Autodesk Fusion 360 part; units mm, degrees
(part 6 of 7)
  line L382 (70.9, -77.2) -> (47.4908, -77.2)
  arc A190 (46.4092, -77.2) -> (47.4908, -77.2) centre (46.95, -80.1) ccw
  line L383 (46.4092, -77.2) -> (23, -77.2)
  line L384 (23, -77.2) -> (23, -81.15)
  arc A191 (18, -81.15) -> (23, -81.15) centre (20.5, -81.15) ccw
  line L385 (27.2, 4.5) -> (27.2, 33.9)
  line L386 (27.2, 33.9) -> (66.7, 33.9)
  line L387 (66.7, 33.9) -> (66.7, 4.5)
  line L388 (66.7, 4.5) -> (27.2, 4.5)
  arc A192 (28.2, 12.5) -> (31.2, 9.5) centre (31.2, 12.5) ccw
  line L389 (31.2, 9.5) -> (62.7, 9.5)
  arc A193 (62.7, 9.5) -> (65.7, 12.5) centre (62.7, 12.5) ccw
  line L390 (65.7, 12.5) -> (65.7, 25.9)
  arc A194 (65.7, 25.9) -> (62.7, 28.9) centre (62.7, 25.9) ccw
  line L391 (62.7, 28.9) -> (31.2, 28.9)
  arc A195 (31.2, 28.9) -> (28.2, 25.9) centre (31.2, 25.9) ccw
  line L392 (28.2, 25.9) -> (28.2, 12.5)
  line L393 (-2, -85.1) -> (106.4, -85.1)
  line L394 (106.4, -85.1) -> (75.9, -85.1)
  line L395 (75.9, -85.1) -> (-2, -85.1)
  line L396 (24.5, -83.65) -> (24.5, -81.15)
  line L397 (24.5, -81.15) -> (24.5, -77.2)
  line L398 (24.5, -77.2) -> (16.5, -77.2)
  line L399 (16.5, -77.2) -> (16.5, -83.65)
  line L400 (16.5, -83.65) -> (-2, -83.65)
  line L401 (-2, -83.65) -> (-2, -3.65)
  line L402 (-2, -3.65) -> (-7, -3.65)
  line L403 (-7, -3.65) -> (-7, 4.1)
  line L404 (-7, 4.1) -> (100.9, 4.1)
  line L405 (100.9, 4.1) -> (100.9, -3.65)
  line L406 (100.9, -3.65) -> (95.9, -3.65)
  line L407 (95.9, -3.65) -> (95.9, -83.65)
  line L408 (95.9, -83.65) -> (24.5, -83.65)
  circle A196 centre (10.06, -44.3) radius 2.5
  circle A197 centre (8, -81.15) radius 1
  circle A198 centre (80.15, -44.4) radius 2.5
  circle A199 centre (-4.5, 1.6) radius 1
  circle A200 centre (73.4, -81.15) radius 1
  circle A201 centre (98.4, 1.6) radius 1
  circle A202 centre (84.4, -5) radius 2.5
  line L409 (16.5, -83.65) -> (-2, -83.65)
  line L410 (-2, -83.65) -> (16.5, -83.65)
  line L411 (27.2, 4.5) -> (66.7, 4.5)
  line L412 (66.7, 4.5) -> (27.2, 4.5)
  line L413 (16.5, -77.2) -> (16.5, -83.65)
  line L414 (16.5, -83.65) -> (16.5, -77.2)
  line L415 (116.4, 35.3) -> (-22.5, 35.3)
  line L416 (-22.5, 35.3) -> (-2.5, 35.3)
  line L417 (-2.5, 35.3) -> (96.4, 35.3)
  line L418 (96.4, 35.3) -> (116.4, 35.3)
  circle A203 centre (10.06, -44.3) radius 2.5
  circle A204 centre (10.06, -44.3) radius 2.5
  line L419 (96.4, 34.3) -> (96.4, 35.3)
  line L420 (96.4, 35.3) -> (-2.5, 35.3)
  line L421 (-2.5, 35.3) -> (-2.5, 34.3)
  line L422 (-2.5, 34.3) -> (-22.5, 34.3)
  arc A205 (-22.5, 34.3) -> (-31.5, 25.3) centre (-22.5, 25.3) ccw
  line L423 (-31.5, 25.3) -> (-31.5, 4.1)
  line L424 (-31.5, 4.1) -> (-25, 4.1)
  line L425 (-25, 4.1) -> (-25, 1.6)
  arc A206 (-23, 4.0495) -> (-25, 1.6) centre (-22.5, 1.6) ccw
  line L426 (-23, 4.0495) -> (-23, 22.8505)
  arc A207 (-22, 22.8505) -> (-23, 22.8505) centre (-22.5, 25.3) ccw
  line L427 (-22, 22.8505) -> (-22, 4.0495)
  arc A208 (-20, 1.6) -> (-22, 4.0495) centre (-22.5, 1.6) ccw
  line L428 (-20, 1.6) -> (-20, 2)
  line L429 (-20, 2) -> (-7, 2)
  line L430 (-7, 2) -> (-7, 4.1)
  line L431 (-7, 4.1) -> (-4.5, 4.1)
  line L432 (-4.5, 4.1) -> (-2, 4.1)
  line L433 (-2, 4.1) -> (0, 4.1)
  line L434 (0, 4.1) -> (0, 5.7)
  arc A209 (13.4164, 23.7) -> (0, 5.7) centre (0, 19.7) ccw
  line L435 (13.4164, 23.7) -> (27.2, 23.7)
  line L436 (27.2, 23.7) -> (27.2, 33.9)
  line L437 (27.2, 33.9) -> (66.7, 33.9)
  line L438 (66.7, 33.9) -> (66.7, 23.7)
  line L439 (66.7, 23.7) -> (80.4836, 23.7)
  arc A210 (93.9, 5.7) -> (80.4836, 23.7) centre (93.9, 19.7) ccw
  line L440 (93.9, 5.7) -> (93.9, 4.1)
  line L441 (93.9, 4.1) -> (95.9, 4.1)
  line L442 (95.9, 4.1) -> (98.4, 4.1)
  line L443 (98.4, 4.1) -> (100.9, 4.1)
  line L444 (100.9, 4.1) -> (100.9, 2)
  line L445 (100.9, 2) -> (113.9322, 2)
  arc A211 (115.9, 4.0495) -> (113.9322, 2) centre (116.4, 1.6) ccw
  line L446 (115.9, 4.0495) -> (115.9, 22.8505)
  arc A212 (116.9, 22.8505) -> (115.9, 22.8505) centre (116.4, 25.3) ccw
  line L447 (116.9, 22.8505) -> (116.9, 4.0495)
  arc A213 (118.9, 1.6) -> (116.9, 4.0495) centre (116.4, 1.6) ccw
  line L448 (118.9, 1.6) -> (118.9, 4.1)
  line L449 (118.9, 4.1) -> (125.4, 4.1)
  line L450 (125.4, 4.1) -> (125.4, 25.3)
  arc A214 (125.4, 25.3) -> (116.4, 34.3) centre (116.4, 25.3) ccw
  line L451 (116.4, 34.3) -> (96.4, 34.3)
  line L452 (-2, -3.65) -> (-2, -83.65)
  line L453 (-2, -83.65) -> (-2, -3.65)
  line L454 (24.5, -81.15) -> (24.5, -77.2)
  line L455 (24.5, -77.2) -> (24.5, -81.15)
  line L456 (-12.5, -85.1) -> (-12.5, -84.1)
  line L457 (-12.5, -84.1) -> (106.4, -84.1)
  line L458 (106.4, -85.1) -> (106.4, -84.1)
  line L459 (106.4, -85.1) -> (-2, -85.1)
  line L460 (-2, -85.1) -> (-12.5, -85.1)
  line L461 (66.7, 33.9) -> (27.2, 33.9)
  line L462 (27.2, 33.9) -> (66.7, 33.9)
  circle A215 centre (-4.5, 1.6) radius 1
  circle A216 centre (-4.5, 1.6) radius 1
  arc A217 (83.1181, 15.7) -> (83.1181, 23.7) centre (93.9, 19.7) ccw
  line L463 (83.1181, 23.7) -> (66.7, 23.7)
  line L464 (66.7, 23.7) -> (66.7, 15.7)
  line L465 (66.7, 15.7) -> (83.1181, 15.7)
  arc A218 (102.9, 18.7) -> (102.9, 20.7) centre (102.9, 19.7) ccw
  line L466 (102.9, 18.7) -> (84.9, 18.7)
  arc A219 (84.9, 20.7) -> (84.9, 18.7) centre (84.9, 19.7) ccw
  line L467 (84.9, 20.7) -> (102.9, 20.7)
  arc A220 (98.9004, 26.7) -> (98.9, 28.7) centre (98.9, 27.7) ccw
  line L468 (98.9004, 26.7) -> (88.8996, 26.7)
  arc A221 (88.9, 28.7) -> (88.8996, 26.7) centre (88.9, 27.7) ccw
  line L469 (88.9, 28.7) -> (98.9, 28.7)
  arc A222 (102.0652, 22.7) -> (102.0652, 24.7) centre (102.0652, 23.7) ccw
  line L470 (102.0652, 22.7) -> (85.7348, 22.7)
  arc A223 (85.7348, 24.7) -> (85.7348, 22.7) centre (85.7348, 23.7) ccw
  line L471 (85.7348, 24.7) -> (102.0652, 24.7)
  line L472 (102.0652, 14.7) -> (85.7348, 14.7)
  arc A224 (85.7348, 16.7) -> (85.7348, 14.7) centre (85.7348, 15.7) ccw
  line L473 (85.7348, 16.7) -> (102.0652, 16.7)
  arc A225 (102.0652, 14.7) -> (102.0652, 16.7) centre (102.0652, 15.7) ccw
  line L474 (88.8996, 12.7) -> (98.8996, 12.7)
  arc A226 (98.9, 10.7) -> (98.8996, 12.7) centre (98.9, 11.7) ccw
  line L475 (98.9, 10.7) -> (88.9, 10.7)
  arc A227 (88.8996, 12.7) -> (88.9, 10.7) centre (88.9, 11.7) ccw
  line L476 (-23.188, -62.3239) -> (-23.188, -59.3239)
  arc A228 (-20.188, -59.3239) -> (-23.188, -59.3239) centre (-21.688, -59.3239) ccw
  line L477 (-20.188, -59.3239) -> (-20.188, -62.3239)
  arc A229 (-23.188, -62.3239) -> (-20.188, -62.3239) centre (-21.688, -62.3239) ccw
  circle A230 centre (-10.8119, -62.3239) radius 1.5
  line L478 (-2, -24.9) -> (-8, -24.9)
  line L479 (-8, -24.9) -> (-8, -7.9)
  line L480 (-8, -7.9) -> (-13, -7.9)
  line L481 (-13, -7.9) -> (-13, -13.9)
  line L482 (-13, -13.9) -> (-25, -13.9)
  line L483 (-25, -13.9) -> (-25, -24.9)
  line L484 (-25, -24.9) -> (-30.5, -24.9)
  line L485 (-30.5, -24.9) -> (-30.5, -25.9)
  line L486 (-30.5, -25.9) -> (-31.5, -25.9)
  line L487 (-31.5, -25.9) -> (-31.5, 4.1)
  line L488 (-31.5, 4.1) -> (-32.5, 4.1)
  line L489 (-32.5, 4.1) -> (-32.5, -25.2)
  line L490 (-32.5, -25.2) -> (-32.5, -65.1)
  arc A231 (-32.5, -65.1) -> (-12.5, -85.1) centre (-12.5, -65.1) ccw
  line L491 (-12.5, -85.1) -> (-2, -85.1)
  line L492 (-2, -85.1) -> (-2, -24.9)
  arc A232 (-9.5307, -48.3426) -> (-9.5307, -34.5574) centre (-10.1676, -41.45) ccw
  arc A233 (-22.9827, -48.1827) -> (-9.5307, -48.3426) centre (-16.25, -47.7) ccw
  arc A234 (-22.9827, -34.7173) -> (-22.9827, -48.1827) centre (-22.5, -41.45) ccw
  arc A235 (-9.5307, -34.5574) -> (-22.9827, -34.7173) centre (-16.25, -35.2) ccw
  circle A236 centre (-16.25, -62.1) radius 2.5
  line L493 (-14, -21.7213) -> (-14, -21.5571)
  arc A237 (-18.6299, -19.9) -> (-14, -21.5571) centre (-16.1626, -20.3028) ccw
  line L494 (-18.6299, -19.9) -> (-18.6563, -19.9)
  arc A238 (-18.6098, -19.7916) -> (-18.6563, -19.9) centre (-16.3363, -20.8316) ccw
  arc A239 (-13.8891, -21.3427) -> (-18.6098, -19.7916) centre (-16.1626, -20.3028) ccw
  arc A240 (-14, -21.7213) -> (-13.8891, -21.3427) centre (-16.3363, -20.8316) ccw
  line L495 (-28.5, -61.1) -> (-28.5, -52.1)
  line L496 (-28.5, -52.1) -> (-27.5, -52.1)
  line L497 (-27.5, -52.1) -> (-27.5, -62.1)
  line L498 (-27.5, -62.1) -> (-24.5, -65.1)
  line L499 (-24.5, -65.1) -> (-19.8023, -65.1)
  arc A241 (-19.8023, -65.1) -> (-12.5, -72.4023) centre (-12.5, -65.1) ccw
  line L500 (-12.5, -72.4023) -> (-12.5, -77.1)
  line L501 (-12.5, -77.1) -> (-6.5, -83.1)
  line L502 (-6.5, -83.1) -> (-6.5, -84.1)
  line L503 (-6.5, -84.1) -> (-12.5, -84.1)
  arc A242 (-31.5, -65.1) -> (-12.5, -84.1) centre (-12.5, -65.1) ccw
  line L504 (-31.5, -65.1) -> (-31.5, -59.1)
  line L505 (-31.5, -59.1) -> (-30.5, -59.1)
  line L506 (-30.5, -59.1) -> (-28.5, -61.1)
  line L507 (-5, -57) -> (-5, -75)
  line L508 (-5, -75) -> (-6, -75)
  line L509 (-6, -75) -> (-6, -57)
  line L510 (-6, -57) -> (-5, -57)
  line L511 (-2, -71.1) -> (-2, -27.1)
  line L512 (-2, -27.1) -> (-2, -0.9)
  line L513 (-2, -0.9) -> (-2, -1.9)
  line L514 (-2, -1.9) -> (-2, -6.9)
  line L515 (-2, -6.9) -> (-2, -7.9)
  line L516 (-2, -7.9) -> (-2, -12.9)
  line L517 (-2, -12.9) -> (-2, -13.9)
  line L518 (-2, -13.9) -> (-2, -18.9)
  line L519 (-2, -18.9) -> (-2, -24.9)
  line L520 (-2, -24.9) -> (-2, -85.1)
  line L521 (-2, -85.1) -> (-2, -77.2)
  line L522 (-2, -77.2) -> (-2, -71.1)
  line L523 (-32.5, -25.2) -> (-31.5, -25.2)
  line L524 (-32.5, -25.2) -> (-32.5, 4.1)
  line L525 (-32.5, 4.1) -> (-32.5, 25.3)
  line L526 (-32.5, 25.3) -> (-31.5, 25.3)
  line L527 (-31.5, 25.3) -> (-31.5, -25.2)
  line L528 (31.2, 9.5) -> (62.7, 9.5)
  line L529 (62.7, 9.5) -> (31.2, 9.5)
  spline S8 degree 3 poles (-32.8222, -7.2428) (-33.1865, -8.6078) (-33.3665, -10.0329) (-33.3734, -12.8887) (-33.1935, -14.3424) (-32.8222, -15.7336) knots 0 0 0 0 0.423819 0.423819 0.855786 0.855786 0.855786 0.855786
  spline S9 degree 3 poles (-32.5, -4.7455) (-32.5, -5.4939) (-32.584, -6.2471) (-32.7761, -7.0646) (-32.7985, -7.1539) (-32.8222, -7.2428) knots 0 0 0 0 0.224513 0.224513 0.252112 0.252112 0.252112 0.252112
  line L530 (-32.5, -4.7455) -> (-32.5, 4.1)
  line L531 (-32.5, 4.1) -> (-31.5, 4.1)
  line L532 (-31.5, 4.1) -> (-31.5, -25.9)
  line L533 (-31.5, -25.9) -> (-31.5, -59.1)
  line L534 (-31.5, -59.1) -> (-31.5, -65.1)
  line L535 (-31.5, -65.1) -> (-32.5, -65.1)
  line L536 (-32.5, -65.1) -> (-32.5, -25.2)
  line L537 (-32.5, -25.2) -> (-32.5, -18.2308)
  spline S10 degree 3 poles (-32.8222, -15.7336) (-32.7995, -15.8187) (-32.778, -15.9042) (-32.5849, -16.7214) (-32.5, -17.4786) (-32.5, -18.2308) knots 0.187001 0.187001 0.187001 0.187001 0.213353 0.213353 0.43842 0.43842 0.43842 0.43842
  arc A243 (85.2397, 8.7) -> (93.9, 5.7) centre (93.9, 19.7) ccw
  line L538 (85.2397, 8.7) -> (66.7, 8.7)
  line L539 (66.7, 8.7) -> (66.7, 4.1)
  line L540 (66.7, 4.1) -> (93.9, 4.1)
  line L541 (93.9, 4.1) -> (93.9, 5.7)
  line L542 (-7, 4.1) -> (-7, -3.65)
  line L543 (-7, -3.65) -> (-7, 4.1)
  line L544 (-31.5, -25.9) -> (-31.5, 4.1)
  line L545 (-31.5, 4.1) -> (-31.5, -65.1)
  line L546 (-31.5, -65.1) -> (-31.5, -59.1)
  line L547 (-31.5, -59.1) -> (-31.5, -25.9)
  arc A244 (80.4836, 15.7) -> (85.2397, 8.7) centre (93.9, 19.7) ccw
  arc A245 (85.2397, 8.7) -> (93.9, 5.7) centre (93.9, 19.7) ccw
  arc A246 (93.9, 5.7) -> (80.4836, 23.7) centre (93.9, 19.7) ccw
  arc A247 (80.4836, 15.7) -> (80.4836, 23.7) centre (93.9, 19.7) ccw
  line L548 (-32.5, -18.2308) -> (-32.5, 11.7692)
  line L549 (-32.5, -18.2308) -> (-32.5, -25.2)
  line L550 (-32.5, -25.2) -> (-32.5, 11.7692)
  spline S11 degree 3 poles (-32.8222, 14.2664) (-33.1865, 15.6314) (-33.3665, 17.0565) (-33.3734, 19.9123) (-33.1935, 21.3661) (-32.8222, 22.7572) knots 0 0 0 0 0.423819 0.423819 0.855786 0.855786 0.855786 0.855786
  spline S12 degree 3 poles (-32.5, 11.7692) (-32.5, 12.5174) (-32.584, 13.2705) (-32.776, 14.088) (-32.7984, 14.1774) (-32.8222, 14.2664) knots 0 0 0 0 0.224479 0.224479 0.252112 0.252112 0.252112 0.252112
  line L551 (-32.5, 11.7692) -> (-32.5, -25.2)
  line L552 (-32.5, -25.2) -> (-32.5, -65.1)
  line L553 (-32.5, -65.1) -> (-31.5, -65.1)
  line L554 (-31.5, -65.1) -> (-31.5, 4.1)
  line L555 (-31.5, 4.1) -> (-31.5, 25.3)
  arc A248 (-22.5, 34.3) -> (-31.5, 25.3) centre (-22.5, 25.3) ccw
  line L556 (-22.5, 34.3) -> (-2.5, 34.3)
  line L557 (-2.5, 34.3) -> (-2.5, 35.3)
  line L558 (-2.5, 35.3) -> (-22.5, 35.3)
  arc A249 (-22.5, 35.3) -> (-32.5, 25.3) centre (-22.5, 25.3) ccw
  line L559 (-32.5, 25.3) -> (-32.5, 25.2545)
  spline S13 degree 3 poles (-32.8222, 22.7572) (-32.7994, 22.8424) (-32.7779, 22.928) (-32.5849, 23.7452) (-32.5, 24.5023) (-32.5, 25.2545) knots 0.187001 0.187001 0.187001 0.187001 0.213377 0.213377 0.43842 0.43842 0.43842 0.43842
  line L560 (100.9, -3.65) -> (100.9, 4.1)
  line L561 (100.9, 4.1) -> (100.9, -3.65)
  line L562 (95.9, -3.65) -> (100.9, -3.65)
  line L563 (100.9, -3.65) -> (95.9, -3.65)
  line L564 (80.4836, 23.7) -> (66.7, 23.7)
  line L565 (66.7, 23.7) -> (83.1181, 23.7)
  line L566 (83.1181, 23.7) -> (80.4836, 23.7)
  arc A250 (10.7819, 23.7) -> (10.7819, 15.7) centre (0, 19.7) ccw
  line L567 (10.7819, 15.7) -> (27.2, 15.7)
  line L568 (27.2, 15.7) -> (27.2, 23.7)
  line L569 (27.2, 23.7) -> (10.7819, 23.7)
  arc A251 (-5.0004, 12.7) -> (-5, 10.7) centre (-5, 11.7) ccw
  line L570 (-5.0004, 12.7) -> (5.0004, 12.7)
  arc A252 (5, 10.7) -> (5.0004, 12.7) centre (5, 11.7) ccw
  line L571 (5, 10.7) -> (-5, 10.7)
  arc A253 (-5, 28.7) -> (-5.0004, 26.7) centre (-5, 27.7) ccw
  line L572 (-5, 28.7) -> (5, 28.7)
  arc A254 (4.9996, 26.7) -> (5, 28.7) centre (5, 27.7) ccw
  line L573 (4.9996, 26.7) -> (-5.0004, 26.7)
  line L574 (-8.1652, 24.7) -> (8.1652, 24.7)
  arc A255 (8.1652, 22.7) -> (8.1652, 24.7) centre (8.1652, 23.7) ccw
  line L575 (8.1652, 22.7) -> (-8.1652, 22.7)
  arc A256 (-8.1652, 24.7) -> (-8.1652, 22.7) centre (-8.1652, 23.7) ccw
  line L576 (8.1652, 14.7) -> (-8.1652, 14.7)
  arc A257 (-8.1652, 16.7) -> (-8.1652, 14.7) centre (-8.1652, 15.7) ccw
  line L577 (-8.1652, 16.7) -> (8.1652, 16.7)
  arc A258 (8.1652, 14.7) -> (8.1652, 16.7) centre (8.1652, 15.7) ccw
  arc A259 (9, 18.7) -> (9, 20.7) centre (9, 19.7) ccw
  line L578 (9, 18.7) -> (-9, 18.7)
  arc A260 (-9, 20.7) -> (-9, 18.7) centre (-9, 19.7) ccw
  line L579 (-9, 20.7) -> (9, 20.7)
  line L580 (126.4, -18.1364) -> (126.4, 11.7754)
  line L581 (126.4, 11.7754) -> (126.4, -65.1)
  line L582 (126.4, -65.1) -> (126.4, 25.3)
  line L583 (126.4, 25.3) -> (126.4, 25.2545)
  line L584 (126.4, 25.2545) -> (126.4, -4.7455)
  line L585 (126.4, -4.7455) -> (126.4, -18.1364)
  line L586 (-32.5, -25.2) -> (-31.5, -25.2)
  line L587 (-31.5, -25.2) -> (-31.5, -65.1)
  line L588 (-32.5, -65.1) -> (-31.5, -65.1)
  line L589 (-32.5, -65.1) -> (-32.5, -25.2)
  arc A261 (-10.0022, -47.8655) -> (-10.0022, -35.0345) centre (-10.1676, -41.45) ccw
  arc A262 (-10.0022, -47.8655) -> (-10.0022, -35.0345) centre (-10.1676, -41.45) ccw
  line L590 (-12.5, -85.1) -> (-12.5, -84.1)
  arc A263 (-32.5, -65.1) -> (-12.5, -85.1) centre (-12.5, -65.1) ccw
  line L591 (-32.5, -65.1) -> (-31.5, -65.1)
  arc A264 (-31.5, -65.1) -> (-12.5, -84.1) centre (-12.5, -65.1) ccw
  circle A265 centre (110.15, -33.95) radius 3.85
  circle A266 centre (110.15, -33.95) radius 3.85
  line L592 (-7, -44.7) -> (-7, -38.2)
  line L593 (-7, -38.2) -> (-7, -44.7)
  line L594 (75.9, -77.2) -> (95.9, -77.2)
  line L595 (95.9, -77.2) -> (75.9, -77.2)
  arc A267 (-22.5, -35.2) -> (-22.5, -47.7) centre (-22.5, -41.45) ccw
  arc A268 (-22.5, -35.2) -> (-22.5, -47.7) centre (-22.5, -41.45) ccw
  arc A269 (-20.188, -59.3239) -> (-23.188, -59.3239) centre (-21.688, -59.3239) ccw
  arc A270 (-20.188, -59.3239) -> (-23.188, -59.3239) centre (-21.688, -59.3239) ccw
  arc A271 (-22.5, -47.7) -> (-10.0022, -47.8655) centre (-16.25, -47.7) ccw
  arc A272 (-22.5, -47.7) -> (-10.0022, -47.8655) centre (-16.25, -47.7) ccw
  spline S14 degree 3 poles (126.7227, 22.7553) (127.0885, 21.3861) (127.2684, 19.9562) (127.2724, 17.1016) (127.0924, 15.654) (126.7221, 14.2685) knots 0 0 0 0 0.425176 0.425176 0.855407 0.855407 0.855407 0.855407
  ellipse E4 centre (131.4, 25.2545) end of major axis (131.4, 18.1834) minor radius 5 (126.4, 25.2545) -> (126.7227, 22.7553) ccw
  line L596 (126.4, 25.2545) -> (126.4, 25.3)
  arc A273 (126.4, 25.3) -> (116.4, 35.3) centre (116.4, 25.3) ccw
  line L597 (116.4, 35.3) -> (96.4, 35.3)
  line L598 (96.4, 35.3) -> (96.4, 34.3)
  line L599 (96.4, 34.3) -> (116.4, 34.3)
  arc A274 (125.4, 25.3) -> (116.4, 34.3) centre (116.4, 25.3) ccw
  line L600 (125.4, 25.3) -> (125.4, 4.1)
  line L601 (125.4, 4.1) -> (125.4, -65.1)
  line L602 (125.4, -65.1) -> (126.4, -65.1)
  line L603 (126.4, -65.1) -> (126.4, 11.7754)
  ellipse E5 centre (131.4, 11.7754) end of major axis (131.4, 18.8361) minor radius 5 (126.7221, 14.2685) -> (126.4, 11.7754) ccw
  circle A275 centre (110.15, -33.95) radius 3.85
  line L604 (112.3409, -38.5) -> (107.9591, -38.5)
  arc A276 (107.5299, -38.2671) -> (107.9591, -38.5) centre (110.15, -33.95) ccw
  line L605 (107.5299, -38.2671) -> (107.1448, -38.6523)
  line L606 (107.1448, -38.6523) -> (105.4477, -36.9552)
  line L607 (105.4477, -36.9552) -> (105.8329, -36.5701)
  arc A277 (107.9591, -29.4) -> (105.8329, -36.5701) centre (110.15, -33.95) ccw
  line L608 (107.9591, -29.4) -> (112.3409, -29.4)
  arc A278 (112.3409, -38.5) -> (112.3409, -29.4) centre (110.15, -33.95) ccw
  line L609 (24.5, -81.15) -> (24.5, -83.65)
  line L610 (24.5, -83.65) -> (95.9, -83.65)
  line L611 (95.9, -83.65) -> (95.9, -3.65)
  line L612 (95.9, -3.65) -> (100.9, -3.65)
  line L613 (100.9, -3.65) -> (100.9, 4.1)
  line L614 (100.9, 4.1) -> (-7, 4.1)
  line L615 (-7, 4.1) -> (-7, -3.65)
  line L616 (-7, -3.65) -> (-2, -3.65)
  line L617 (-2, -3.65) -> (-2, -83.65)
  line L618 (-2, -83.65) -> (16.5, -83.65)
  line L619 (16.5, -83.65) -> (16.5, -77.2)
  line L620 (16.5, -77.2) -> (24.5, -77.2)
  line L621 (24.5, -77.2) -> (24.5, -81.15)
  circle A279 centre (84.4, -5) radius 2.5
  circle A280 centre (98.4, 1.6) radius 1
  circle A281 centre (73.4, -81.15) radius 1
  circle A282 centre (-4.5, 1.6) radius 1
  circle A283 centre (80.15, -44.4) radius 2.5
  circle A284 centre (8, -81.15) radius 1
  circle A285 centre (10.06, -44.3) radius 2.5
  arc A286 (-10.0022, -47.8655) -> (-10.0022, -35.0345) centre (-10.1676, -41.45) ccw
  arc A287 (-22.5, -47.7) -> (-10.0022, -47.8655) centre (-16.25, -47.7) ccw
  arc A288 (-22.5, -35.2) -> (-22.5, -47.7) centre (-22.5, -41.45) ccw
  arc A289 (-10.0022, -35.0345) -> (-22.5, -35.2) centre (-16.25, -35.2) ccw
  arc A290 (-9.5307, -34.5574) -> (-22.9827, -34.7173) centre (-16.25, -35.2) ccw
  arc A291 (-22.9827, -34.7173) -> (-22.9827, -48.1827) centre (-22.5, -41.45) ccw
  arc A292 (-22.9827, -48.1827) -> (-9.5307, -48.3426) centre (-16.25, -47.7) ccw
  arc A293 (-9.5307, -48.3426) -> (-9.5307, -34.5574) centre (-10.1676, -41.45) ccw
  line L622 (-25, -24.9) -> (-25, -13.9)
  line L623 (-25, -13.9) -> (-13, -13.9)
  line L624 (-13, -13.9) -> (-13, -7.9)
  line L625 (-13, -7.9) -> (-8, -7.9)
  line L626 (-8, -7.9) -> (-8, -24.9)
  line L627 (-8, -24.9) -> (-2, -24.9)
  line L628 (-2, -24.9) -> (-2, -18.9)
  line L629 (-2, -18.9) -> (-6.9926, -18.9)
  line L630 (-6.9926, -18.9) -> (-6.9864, -13.9)
  line L631 (-6.9864, -13.9) -> (-2, -13.9)
  line L632 (-2, -13.9) -> (-2, -12.9)
  line L633 (-2, -12.9) -> (-6.9852, -12.9)
  line L634 (-6.9852, -12.9) -> (-6.979, -7.9)
  line L635 (-6.979, -7.9) -> (-2, -7.9)
  line L636 (-2, -7.9) -> (-2, -6.9)
  line L637 (-2, -6.9) -> (-6.9778, -6.9)
  line L638 (-6.9778, -6.9) -> (-6.9716, -1.9)
  line L639 (-6.9716, -1.9) -> (-2, -1.9)
  line L640 (-2, -1.9) -> (-2, -0.9)
  line L641 (-2, -0.9) -> (-4.5, -0.9)
  arc A294 (-6.9678, 1.2) -> (-4.5, -0.9) centre (-4.5, 1.6) ccw
  line L642 (-6.9678, 1.2) -> (-20.0322, 1.2)
  arc A295 (-22.4996, -0.9) -> (-20.0322, 1.2) centre (-22.5, 1.6) ccw
  line L643 (-22.4996, -0.9) -> (-25, -0.9)
  line L644 (-25, -0.9) -> (-25, 1.6)
  line L645 (-25, 1.6) -> (-25, 4.1)
  line L646 (-25, 4.1) -> (-26, 4.1)
  line L647 (-26, 4.1) -> (-26, -0.9)
  line L648 (-26, -0.9) -> (-30.5, -0.9)
  line L649 (-30.5, -0.9) -> (-30.5, 4.1)
  line L650 (-30.5, 4.1) -> (-31.5, 4.1)
  line L651 (-31.5, 4.1) -> (-31.5, -25.9)
  line L652 (-31.5, -25.9) -> (-30.5, -25.9)
  line L653 (-30.5, -25.9) -> (-30.5, -24.9)
  line L654 (-30.5, -24.9) -> (-25, -24.9)
  line L655 (-20, -6.9) -> (-25, -6.9)
  line L656 (-25, -6.9) -> (-25, -1.9)
  line L657 (-25, -1.9) -> (-20, -1.9)
  line L658 (-20, -1.9) -> (-20, -6.9)
  line L659 (-26, -18.9) -> (-30.5, -18.9)
  line L660 (-30.5, -18.9) -> (-30.5, -13.9)
  line L661 (-30.5, -13.9) -> (-26, -13.9)
  line L662 (-26, -13.9) -> (-26, -18.9)
  line L663 (-26, -6.9) -> (-30.5, -6.9)
  line L664 (-30.5, -6.9) -> (-30.5, -1.9)
  line L665 (-30.5, -1.9) -> (-26, -1.9)
  line L666 (-26, -1.9) -> (-26, -6.9)
  line L667 (-19, -6.9) -> (-19, -1.9)
  line L668 (-19, -1.9) -> (-14, -1.9)
  line L669 (-14, -1.9) -> (-14, -6.9)
  line L670 (-14, -6.9) -> (-19, -6.9)
  line L671 (66.7, 15.7) -> (66.7, 23.7)
  line L672 (66.7, 23.7) -> (66.7, 33.9)
  line L673 (66.7, 33.9) -> (66.7, 30.4)
  line L674 (66.7, 30.4) -> (66.7, 10)
  line L675 (66.7, 10) -> (66.7, 4.1)
  line L676 (66.7, 4.1) -> (66.7, 8.7)
  line L677 (66.7, 8.7) -> (66.7, 15.7)
  line L678 (10.7819, 23.7) -> (13.4164, 23.7)
  arc A296 (13.4164, 23.7) -> (13.4164, 15.7) centre (0, 19.7) ccw
  line L679 (13.4164, 15.7) -> (10.7819, 15.7)
  arc A297 (10.7819, 23.7) -> (10.7819, 15.7) centre (0, 19.7) ccw
  line L680 (126.4, -65.1) -> (125.4, -65.1)
  line L681 (125.4, -65.1) -> (125.4, 25.3)
  line L682 (126.4, 25.3) -> (125.4, 25.3)
  line L683 (126.4, 25.3) -> (126.4, -65.1)
  arc A298 (5.5, -81.15) -> (10.5, -81.15) centre (8, -81.15) ccw
  arc A299 (5.5, -81.15) -> (10.5, -81.15) centre (8, -81.15) ccw
  line L684 (95.9, -71.1) -> (95.9, -77.2)
  line L685 (95.9, -77.2) -> (95.9, -25.9)
  line L686 (95.9, -25.9) -> (95.9, -24.9)
  line L687 (95.9, -24.9) -> (95.9, -0.9)
  line L688 (95.9, -0.9) -> (95.9, -27.1)
  line L689 (95.9, -27.1) -> (95.9, -71.1)
  line L690 (24.5, -83.65) -> (95.9, -83.65)
  line L691 (95.9, -83.65) -> (24.5, -83.65)
  line L692 (93.9, -71.1) -> (93.9, -27.1)
  line L693 (93.9, -27.1) -> (93.9, 4.1)
  line L694 (93.9, 4.1) -> (93.9, 5.7)
  line L695 (93.9, 5.7) -> (93.9, 4.1)
  line L696 (93.9, 4.1) -> (93.9, -75.1)
  line L697 (93.9, -75.1) -> (93.9, -71.1)
  line L698 (5.5, -77.2) -> (-2, -77.2)
  line L699 (-2, -77.2) -> (5.5, -77.2)
  line L700 (70.9, -77.2) -> (70.9, -81.15)
  line L701 (70.9, -81.15) -> (70.9, -77.2)
  line L702 (-30.5, -25.9) -> (-30.5, -24.9)
  line L703 (-30.5, -24.9) -> (-30.5, -25.9)
  arc A300 (70.9, -81.15) -> (75.9, -81.15) centre (73.4, -81.15) ccw
  arc A301 (70.9, -81.15) -> (75.9, -81.15) centre (73.4, -81.15) ccw
  line L704 (95.9, -83.65) -> (95.9, -3.65)
  line L705 (95.9, -3.65) -> (95.9, -83.65)
  line L706 (125.4, 4.1) -> (125.4, -65.1)
  line L707 (125.4, -65.1) -> (125.4, 4.1)
  arc A302 (-9.5307, -48.3426) -> (-9.5307, -34.5574) centre (-10.1676, -41.45) ccw
  arc A303 (-9.5307, -48.3426) -> (-9.5307, -34.5574) centre (-10.1676, -41.45) ccw
  arc A304 (13.4164, 23.7) -> (0, 5.7) centre (0, 19.7) ccw
  arc A305 (0, 5.7) -> (8.6603, 8.7) centre (0, 19.7) ccw
  arc A306 (8.6603, 8.7) -> (13.4164, 15.7) centre (0, 19.7) ccw
  arc A307 (13.4164, 23.7) -> (13.4164, 15.7) centre (0, 19.7) ccw
  line L708 (10.5, -81.15) -> (10.5, -77.2)
  line L709 (10.5, -77.2) -> (10.5, -81.15)
  line L710 (-31.5, -25.9) -> (-30.5, -25.9)
  line L711 (-30.5, -25.9) -> (-31.5, -25.9)
  circle A308 centre (8, -81.15) radius 0.4
  line L712 (80.4836, 15.7) -> (66.7, 15.7)
  line L713 (66.7, 15.7) -> (66.7, 8.7)
  line L714 (66.7, 8.7) -> (85.2397, 8.7)
  arc A309 (80.4836, 15.7) -> (85.2397, 8.7) centre (93.9, 19.7) ccw
  circle A310 centre (8, -81.15) radius 0.4
  circle A311 centre (8, -81.15) radius 0.4
  line L715 (-27.5, -52.1) -> (-28.5, -52.1)
  line L716 (-28.5, -52.1) -> (-27.5, -52.1)
  line L717 (80.4836, 15.7) -> (83.1181, 15.7)
  line L718 (83.1181, 15.7) -> (66.7, 15.7)
  line L719 (66.7, 15.7) -> (80.4836, 15.7)
  line L720 (70.9, -77.2) -> (47.4908, -77.2)
  line L721 (47.4908, -77.2) -> (70.9, -77.2)
  line L722 (93.9, -27.1) -> (93.9, -71.1)
  line L723 (93.9, -71.1) -> (95.9, -71.1)
  line L724 (95.9, -71.1) -> (95.9, -27.1)
  line L725 (95.9, -27.1) -> (93.9, -27.1)
  line L726 (-22.5, 34.3) -> (-2.5, 34.3)
  line L727 (-2.5, 34.3) -> (-22.5, 34.3)
  circle A312 centre (73.4, -81.15) radius 0.4
  circle A313 centre (73.4, -81.15) radius 0.4
  arc A314 (10.7819, 23.7) -> (10.7819, 15.7) centre (0, 19.7) ccw
  arc A315 (10.7819, 23.7) -> (10.7819, 15.7) centre (0, 19.7) ccw
  arc A316 (-10.0022, -35.0345) -> (-22.5, -35.2) centre (-16.25, -35.2) ccw
  arc A317 (-22.5, -35.2) -> (-22.5, -47.7) centre (-22.5, -41.45) ccw
  arc A318 (-22.5, -47.7) -> (-10.0022, -47.8655) centre (-16.25, -47.7) ccw
  arc A319 (-10.0022, -47.8655) -> (-10.0022, -35.0345) centre (-10.1676, -41.45) ccw
  arc A320 (-13, -47.5324) -> (-10.1676, -44.7) centre (-16.25, -41.45) ccw
  line L728 (-13, -47.5324) -> (-13, -50.7)
  line L729 (-13, -50.7) -> (-19.5, -50.7)
  line L730 (-19.5, -50.7) -> (-19.5, -47.5324)
  arc A321 (-22.3324, -44.7) -> (-19.5, -47.5324) centre (-16.25, -41.45) ccw
  line L731 (-22.3324, -44.7) -> (-25.5, -44.7)
  line L732 (-25.5, -44.7) -> (-25.5, -38.2)
  line L733 (-25.5, -38.2) -> (-22.3324, -38.2)
  arc A322 (-19.5, -35.3676) -> (-22.3324, -38.2) centre (-16.25, -41.45) ccw
  line L734 (-19.5, -35.3676) -> (-19.5, -32.2)
  line L735 (-19.5, -32.2) -> (-13, -32.2)
  line L736 (-13, -32.2) -> (-13, -35.3676)
  arc A323 (-10.1676, -38.2) -> (-13, -35.3676) centre (-16.25, -41.45) ccw
  line L737 (-10.1676, -38.2) -> (-7, -38.2)
  line L738 (-7, -38.2) -> (-7, -44.7)
  line L739 (-7, -44.7) -> (-10.1676, -44.7)
  line L740 (-32.5, -25.2) -> (-32.5, -65.1)
  line L741 (-32.5, -65.1) -> (-32.5, -25.2)
  arc A324 (-31.5, -65.1) -> (-12.5, -84.1) centre (-12.5, -65.1) ccw
  arc A325 (-31.5, -65.1) -> (-12.5, -84.1) centre (-12.5, -65.1) ccw
  line L742 (-32.5, -65.1) -> (-31.5, -65.1)
  line L743 (-31.5, -65.1) -> (-32.5, -65.1)
  line L744 (93.9, -27.1) -> (95.9, -27.1)
  line L745 (95.9, -27.1) -> (95.9, -0.9)
  line L746 (95.9, -0.9) -> (98.4, -0.9)
  arc A326 (98.4, -0.9) -> (100.9, 1.6) centre (98.4, 1.6) ccw
  line L747 (100.9, 1.6) -> (100.9, 4.1)
  line L748 (100.9, 4.1) -> (98.4, 4.1)
  line L749 (98.4, 4.1) -> (95.9, 4.1)
  line L750 (95.9, 4.1) -> (93.9, 4.1)
  line L751 (93.9, 4.1) -> (93.9, -27.1)
  circle A327 centre (98.4, 1.6) radius 0.4
  line L752 (5.5, -77.2) -> (5.5, -81.15)
  line L753 (5.5, -81.15) -> (5.5, -77.2)
  circle A328 centre (20.5, -81.15) radius 0.4
  arc A329 (-10.0022, -35.0345) -> (-22.5, -35.2) centre (-16.25, -35.2) ccw
  arc A330 (-10.0022, -35.0345) -> (-22.5, -35.2) centre (-16.25, -35.2) ccw
  line L754 (18, -77.2) -> (10.5, -77.2)
  line L755 (10.5, -77.2) -> (18, -77.2)
  line L756 (-23.188, -62.3239) -> (-23.188, -59.3239)
  line L757 (-23.188, -59.3239) -> (-23.188, -62.3239)
  line L758 (23, -77.2) -> (46.4092, -77.2)
  line L759 (46.4092, -77.2) -> (23, -77.2)
  line L760 (107.9591, -38.5) -> (112.3409, -38.5)
  arc A331 (112.3409, -38.5) -> (112.3409, -29.4) centre (110.15, -33.95) ccw
  line L761 (112.3409, -29.4) -> (107.9591, -29.4)
  arc A332 (107.9591, -29.4) -> (105.8329, -36.5701) centre (110.15, -33.95) ccw
  line L762 (105.8329, -36.5701) -> (105.4477, -36.9552)
  line L763 (105.4477, -36.9552) -> (107.1448, -38.6523)
  line L764 (107.1448, -38.6523) -> (107.5299, -38.2671)
  arc A333 (107.5299, -38.2671) -> (107.9591, -38.5) centre (110.15, -33.95) ccw
  circle A334 centre (110.15, -33.95) radius 3.85
  line L765 (27.2, 23.7) -> (27.2, 15.7)
  line L766 (27.2, 15.7) -> (27.2, 8.7)
  line L767 (27.2, 8.7) -> (27.2, 4.1)
  line L768 (27.2, 4.1) -> (27.2, 10)
  line L769 (27.2, 10) -> (27.2, 30.4)
  line L770 (27.2, 30.4) -> (27.2, 33.9)
  line L771 (27.2, 33.9) -> (27.2, 23.7)
  circle A335 centre (73.4, -81.15) radius 0.4
  line L772 (18, -77.2) -> (18, -81.15)
  line L773 (18, -81.15) -> (18, -77.2)
  line L774 (-20.188, -59.3239) -> (-20.188, -62.3239)
  line L775 (-20.188, -62.3239) -> (-20.188, -59.3239)
  line L776 (8.1652, 22.7) -> (-8.1652, 22.7)
  line L777 (-8.1652, 22.7) -> (8.1652, 22.7)
  line L778 (107.65, -43.95) -> (107.65, -38.95)
  line L779 (107.65, -38.95) -> (112.65, -38.95)
  line L780 (112.65, -38.95) -> (112.65, -43.95)
  line L781 (112.65, -43.95) -> (107.65, -43.95)
  circle A336 centre (-22.5, 1.6) radius 0.4
  circle A337 centre (-22.5, 1.6) radius 0.4
  circle A338 centre (-22.5, 1.6) radius 0.4
  line L782 (112.65, -38.95) -> (107.65, -38.95)
  line L783 (107.65, -38.95) -> (107.65, -43.95)
  line L784 (107.65, -43.95) -> (112.65, -43.95)
  line L785 (112.65, -43.95) -> (112.65, -38.95)
  line L786 (-8.1652, 24.7) -> (8.1652, 24.7)
  line L787 (8.1652, 24.7) -> (-8.1652, 24.7)
  line L788 (-22.5, 35.177) -> (-22.5, 35.3)
  line L789 (-22.5, 35.177) -> (-22.5, 35.3)
  spline S15 degree 3 poles (-32.8222, 14.2664) (-33.1865, 15.6314) (-33.3665, 17.0565) (-33.3734, 19.9123) (-33.1935, 21.3661) (-32.8222, 22.7572) knots 0 0 0 0 0.423819 0.423819 0.855786 0.855786 0.855786 0.855786
  line L790 (-32.8222, 22.7572) -> (-32.8222, -7.2428)
  spline S16 degree 3 poles (-32.8222, -7.2428) (-33.1865, -8.6078) (-33.3665, -10.0329) (-33.3734, -12.8887) (-33.1935, -14.3424) (-32.8222, -15.7336) knots 0 0 0 0 0.423819 0.423819 0.855786 0.855786 0.855786 0.855786
  line L791 (-32.8222, -15.7336) -> (-32.8222, 14.2664)
  circle A339 centre (-22.5, 25.3) radius 0.4
  circle A340 centre (-22.5, 25.3) radius 2.5
  arc A341 (9, 18.7) -> (9, 20.7) centre (9, 19.7) ccw
  arc A342 (9, 18.7) -> (9, 20.7) centre (9, 19.7) ccw
  line L792 (124.4, -24.9) -> (124.4, -25.9)
  line L793 (124.4, -25.9) -> (124.4, -24.9)
  line L794 (-21.5816, -73.1909) -> (-21.2106, -67.0687)
  line L795 (-21.2106, -67.0687) -> (-27.6189, -73.477)
  line L796 (-27.6189, -73.477) -> (-21.5816, -73.1909)
  line L797 (-9, 20.7) -> (9, 20.7)
  line L798 (9, 20.7) -> (-9, 20.7)
  arc A343 (4.9996, 26.7) -> (5, 28.7) centre (5, 27.7) ccw
  arc A344 (4.9996, 26.7) -> (5, 28.7) centre (5, 27.7) ccw
  line L799 (8.1652, 14.7) -> (-8.1652, 14.7)
  line L800 (-8.1652, 14.7) -> (8.1652, 14.7)
  line L801 (118.9, -25.9) -> (118.9, -24.9)
  line L802 (118.9, -24.9) -> (118.9, -25.9)
  line L803 (-32.5, 25.2545) -> (-32.5, -4.7455)
  line L804 (-32.5, 25.2545) -> (-32.5, 25.3)
  line L805 (-32.5, 25.3) -> (-32.5, 4.1)
  line L806 (-32.5, 4.1) -> (-32.5, -4.7455)
  line L807 (-32.8222, -15.7336) -> (-32.8222, 14.2664)
  spline S17 degree 3 poles (-32.8222, -15.7336) (-32.7995, -15.8187) (-32.778, -15.9042) (-32.5849, -16.7214) (-32.5, -17.4786) (-32.5, -18.2308) knots 0.187001 0.187001 0.187001 0.187001 0.213353 0.213353 0.43842 0.43842 0.43842 0.43842
  line L808 (-32.5, -18.2308) -> (-32.5, 11.7692)
  spline S18 degree 3 poles (-32.5, 11.7692) (-32.5, 12.5174) (-32.584, 13.2705) (-32.776, 14.088) (-32.7984, 14.1774) (-32.8222, 14.2664) knots 0 0 0 0 0.224479 0.224479 0.252112 0.252112 0.252112 0.252112
  line L809 (-28.496, -73.3541) -> (-21.2419, -66.1)
  line L810 (-21.2419, -66.1) -> (-30.4722, -66.1)
  arc A345 (-30.4722, -66.1) -> (-28.496, -73.3541) centre (-12.5, -65.1) ccw
  circle A346 centre (117.65, -41.45) radius 3.85
  circle A347 centre (117.65, -41.45) radius 3.85
  line L811 (-32.8222, 22.7572) -> (-32.8222, -7.2428)
  spline S19 degree 3 poles (-32.8222, 22.7572) (-32.7994, 22.8424) (-32.7779, 22.928) (-32.5849, 23.7452) (-32.5, 24.5023) (-32.5, 25.2545) knots 0.187001 0.187001 0.187001 0.187001 0.213377 0.213377 0.43842 0.43842 0.43842 0.43842
  line L812 (-32.5, 25.2545) -> (-32.5, -4.7455)
  spline S20 degree 3 poles (-32.5, -4.7455) (-32.5, -5.4939) (-32.584, -6.2471) (-32.7761, -7.0646) (-32.7985, -7.1539) (-32.8222, -7.2428) knots 0 0 0 0 0.224513 0.224513 0.252112 0.252112 0.252112 0.252112
  circle A348 centre (-22.5, 1.6) radius 2.5
  arc A349 (-22.4996, -0.9) -> (-20.0322, 1.2) centre (-22.5, 1.6) ccw
  arc A350 (-20.0322, 1.2) -> (-20, 1.6) centre (-22.5, 1.6) ccw
  arc A351 (-20, 1.6) -> (-22, 4.0495) centre (-22.5, 1.6) ccw
  arc A352 (-22, 4.0495) -> (-23, 4.0495) centre (-22.5, 1.6) ccw
  arc A353 (-23, 4.0495) -> (-25, 1.6) centre (-22.5, 1.6) ccw
  arc A354 (-25, 1.6) -> (-22.4996, -0.9) centre (-22.5, 1.6) ccw
  line L813 (9, 18.7) -> (-9, 18.7)
  line L814 (-9, 18.7) -> (9, 18.7)
  arc A355 (-9, 20.7) -> (-9, 18.7) centre (-9, 19.7) ccw
  arc A356 (-9, 20.7) -> (-9, 18.7) centre (-9, 19.7) ccw
  line L815 (107.65, -43.95) -> (112.65, -43.95)
  line L816 (112.65, -43.95) -> (107.65, -43.95)
  line L817 (124.4, -25.9) -> (118.9, -25.9)
  line L818 (118.9, -25.9) -> (124.4, -25.9)
  circle A357 centre (117.65, -41.45) radius 3.85
  line L819 (113.1, -43.6409) -> (113.1, -39.2591)
  arc A358 (113.3329, -38.8299) -> (113.1, -39.2591) centre (117.65, -41.45) ccw
  line L820 (113.3329, -38.8299) -> (112.9477, -38.4448)
  line L821 (112.9477, -38.4448) -> (114.6448, -36.7477)
  line L822 (114.6448, -36.7477) -> (115.0299, -37.1329)
  arc A359 (122.2, -39.2591) -> (115.0299, -37.1329) centre (117.65, -41.45) ccw
  line L823 (122.2, -39.2591) -> (122.2, -43.6409)
  arc A360 (113.1, -43.6409) -> (122.2, -43.6409) centre (117.65, -41.45) ccw
  arc A361 (-8.1652, 24.7) -> (-8.1652, 22.7) centre (-8.1652, 23.7) ccw
  arc A362 (-8.1652, 24.7) -> (-8.1652, 22.7) centre (-8.1652, 23.7) ccw
  line L824 (112.65, -43.95) -> (112.65, -38.95)
  line L825 (112.65, -38.95) -> (112.65, -43.95)
  line L826 (-20.0322, 1.2) -> (-6.9678, 1.2)
  arc A363 (-7, 1.6) -> (-6.9678, 1.2) centre (-4.5, 1.6) ccw
  line L827 (-7, 1.6) -> (-7, 2)
  line L828 (-7, 2) -> (-20, 2)
  line L829 (-20, 2) -> (-20, 1.6)
  arc A364 (-20.0322, 1.2) -> (-20, 1.6) centre (-22.5, 1.6) ccw
  line L830 (112.65, -38.95) -> (107.65, -38.95)
  line L831 (107.65, -38.95) -> (112.65, -38.95)
  arc A365 (8.1652, 22.7) -> (8.1652, 24.7) centre (8.1652, 23.7) ccw
  arc A366 (8.1652, 22.7) -> (8.1652, 24.7) centre (8.1652, 23.7) ccw
  line L832 (-20.0322, 1.2) -> (-6.9678, 1.2)
  line L833 (-6.9678, 1.2) -> (-20.0322, 1.2)
  spline S21 degree 3 poles (-24.0635, 35.177) (-24.2027, 35.155) (-24.3417, 35.13) (-25.0454, 34.9877) (-25.6111, 34.8224) (-26.1657, 34.6039) knots 0.177677 0.177677 0.177677 0.177677 0.227456 0.227456 0.429091 0.429091 0.429091 0.429091
  arc A367 (-26.1657, 34.6039) -> (-32.5, 25.3) centre (-22.5, 25.3) ccw
  arc A368 (-22.5, 35.3) -> (-32.5, 25.3) centre (-22.5, 25.3) ccw
  arc A369 (-22.5, 35.3) -> (-24.0635, 35.177) centre (-22.5, 25.3) ccw
  line L834 (-7, 2) -> (-20, 2)
  line L835 (-20, 2) -> (-7, 2)
  line L836 (4.9996, 26.7) -> (-5.0004, 26.7)
  line L837 (-5.0004, 26.7) -> (4.9996, 26.7)
  line L838 (125.4, -65.1) -> (126.4, -65.1)
  line L839 (126.4, -65.1) -> (125.4, -65.1)
  line L840 (-20, 2) -> (-20, 1.6)
  line L841 (-20, 1.6) -> (-20, 2)
  circle A370 centre (102.6547, -56.4453) radius 2.35
  circle A371 centre (102.6547, -56.4453) radius 2.35
  arc A372 (-14, -21.7213) -> (-13.8891, -21.3427) centre (-16.3363, -20.8316) ccw
  arc A373 (-14, -21.7213) -> (-13.8891, -21.3427) centre (-16.3363, -20.8316) ccw
  circle A374 centre (110.15, -48.95) radius 3.85
  line L842 (112.3364, -53.5022) -> (112.3364, -53.5)
  line L843 (112.3364, -53.5) -> (107.9591, -53.5)
  arc A375 (107.9591, -44.4) -> (107.9591, -53.5) centre (110.15, -48.95) ccw
  line L844 (107.9591, -44.4) -> (112.3409, -44.4)
  arc A376 (112.7701, -44.6329) -> (112.3409, -44.4) centre (110.15, -48.95) ccw
  line L845 (112.7701, -44.6329) -> (113.1552, -44.2477)
  line L846 (113.1552, -44.2477) -> (114.8523, -45.9448)
  line L847 (114.8523, -45.9448) -> (114.4671, -46.3299)
  arc A377 (112.3364, -53.5022) -> (114.4671, -46.3299) centre (110.15, -48.95) ccw
  circle A378 centre (-22.5, 25.3) radius 0.4
  arc A379 (-18.6098, -19.7916) -> (-18.6563, -19.9) centre (-16.3363, -20.8316) ccw
  arc A380 (-18.6098, -19.7916) -> (-18.6563, -19.9) centre (-16.3363, -20.8316) ccw
  circle A381 centre (102.6547, -56.4453) radius 2.35
  circle A382 centre (102.6547, -56.4453) radius 5
  line L848 (-22.5, 35.177) -> (-24.0635, 35.177)
  arc A383 (-22.5, 35.3) -> (-24.0635, 35.177) centre (-22.5, 25.3) ccw
  line L849 (-22.5, 35.3) -> (-22.5, 35.177)
  circle A384 centre (-22.5, 1.6) radius 0.4
  circle A385 centre (-22.5, 1.6) radius 2.5
  line L850 (-5, 28.7) -> (5, 28.7)
  line L851 (5, 28.7) -> (-5, 28.7)
  line L852 (106.4, -85.1) -> (106.4, -84.1)
  arc A386 (106.4, -84.1) -> (125.4, -65.1) centre (106.4, -65.1) ccw
  line L853 (126.4, -65.1) -> (125.4, -65.1)
  arc A387 (106.4, -85.1) -> (126.4, -65.1) centre (106.4, -65.1) ccw
  arc A388 (-5, 28.7) -> (-5.0004, 26.7) centre (-5, 27.7) ccw
  arc A389 (-5, 28.7) -> (-5.0004, 26.7) centre (-5, 27.7) ccw
  circle A390 centre (110.15, -48.95) radius 3.85
  circle A391 centre (110.15, -48.95) radius 3.85
  line L854 (-31.5, 4.1) -> (-31.5, -25.9)
  line L855 (-31.5, -25.9) -> (-31.5, 4.1)
  spline S22 degree 3 poles (-26.1657, 34.6039) (-26.5128, 34.4672) (-26.796, 34.2925) (-27.2865, 33.8432) (-27.4579, 33.5817) (-27.6034, 33.268) (-27.6354, 33.1786) (-27.6643, 33.054) (-27.6732, 32.9982) (-27.6666, 32.9257) (-27.6619, 32.9031) (-27.6451, 32.8674) (-27.6355, 32.8538) (-27.6103, 32.831) (-27.5957, 32.8224) (-27.558, 32.8077) (-27.5332, 32.803) (-27.496, 32.8003) (-27.4857, 32.8) (-27.4749, 32.8) knots 0.503021 0.503021 0.503021 0.503021 0.608582 0.608582 0.725176 0.725176 0.775103 0.775103 0.805659 0.805659 0.818798 0.818798 0.828249 0.828249 0.837394 0.837394 0.849434 0.849434 0.853721 0.853721 0.853721 0.853721
  arc A392 (-27.4749, 32.8) -> (-31.5, 25.3) centre (-22.5, 25.3) ccw
  line L856 (-32.5, 25.3) -> (-31.5, 25.3)
  arc A393 (-26.1657, 34.6039) -> (-32.5, 25.3) centre (-22.5, 25.3) ccw
  line L857 (5, 10.7) -> (-5, 10.7)
  line L858 (-5, 10.7) -> (5, 10.7)
  line L859 (-16.4927, 27.4281) -> (-15.2, 27.4281)
  line L860 (-15.2, 27.4281) -> (-16.4927, 27.4281)
  line L861 (-14, -21.5571) -> (-14, -21.7213)
  line L862 (-14, -21.7213) -> (-14, -21.5571)
  arc A394 (5, 10.7) -> (5.0004, 12.7) centre (5, 11.7) ccw
  arc A395 (5, 10.7) -> (5.0004, 12.7) centre (5, 11.7) ccw
  line L863 (-15.2, 27.4281) -> (-15.6347, 27.9403)
  line L864 (-15.6347, 27.9403) -> (-15.2, 27.4281)
  line L865 (-5.0004, 12.7) -> (5.0004, 12.7)
  line L866 (5.0004, 12.7) -> (-5.0004, 12.7)
  arc A396 (-15.6347, 27.9403) -> (-15.8651, 28.0068) centre (-15.8, 27.8) ccw
  arc A397 (-15.6347, 27.9403) -> (-15.8651, 28.0068) centre (-15.8, 27.8) ccw
  arc A398 (-14, -21.5571) -> (-13.8891, -21.3427) centre (-16.1626, -20.3028) ccw
  line L867 (-14, -21.5571) -> (-14, -21.7213)
  arc A399 (-14, -21.7213) -> (-13.8891, -21.3427) centre (-16.3363, -20.8316) ccw
  arc A400 (-5.0004, 12.7) -> (-5, 10.7) centre (-5, 11.7) ccw
  arc A401 (-5.0004, 12.7) -> (-5, 10.7) centre (-5, 11.7) ccw
  circle A402 centre (-16.1626, -20.3028) radius 2.5
  arc A403 (-14, -21.5571) -> (-13.8891, -21.3427) centre (-16.1626, -20.3028) ccw
  arc A404 (-13.8891, -21.3427) -> (-18.6098, -19.7916) centre (-16.1626, -20.3028) ccw
  arc A405 (-18.6098, -19.7916) -> (-18.6299, -19.9) centre (-16.1626, -20.3028) ccw
  arc A406 (-18.6299, -19.9) -> (-14, -21.5571) centre (-16.1626, -20.3028) ccw
  circle A407 centre (117.6453, -56.4453) radius 2.35
  circle A408 centre (117.6453, -56.4453) radius 2.35
  line L868 (93.9, -71.1) -> (95.9, -71.1)
  line L869 (95.9, -71.1) -> (93.9, -71.1)
  line L870 (34.2, 30.4) -> (34.2, 32.4)
  line L871 (34.2, 32.4) -> (34.2, 30.4)
  line L872 (-15.8651, 28.0068) -> (-16.5461, 27.7924)
  line L873 (-16.5461, 27.7924) -> (-15.8651, 28.0068)
  line L874 (-16.2174, 28.8586) -> (-17.0653, 28.0624)
  line L875 (-17.0653, 28.0624) -> (-16.2174, 28.8586)
  arc A409 (-17.8764, 30.7591) -> (-15.9888, 31.4975) centre (-16.1, 29) ccw
  arc A410 (-17.8764, 30.7591) -> (-15.9888, 31.4975) centre (-16.1, 29) ccw
  circle A411 centre (110.15, -62.1) radius 2.5
  circle A412 centre (110.15, -62.1) radius 2.5
  line L876 (-17.0653, 28.0624) -> (-16.4927, 27.4281)
  line L877 (-16.4927, 27.4281) -> (-15.2, 27.4281)
  line L878 (-15.2, 27.4281) -> (-15.6347, 27.9403)
  arc A413 (-15.6347, 27.9403) -> (-15.8651, 28.0068) centre (-15.8, 27.8) ccw
  line L879 (-15.8651, 28.0068) -> (-16.5461, 27.7924)
  line L880 (-16.5461, 27.7924) -> (-16.7087, 27.9725)
  line L881 (-16.7087, 27.9725) -> (-15.4643, 29.0958)
  arc A414 (-15.4643, 29.0958) -> (-16.2174, 28.8586) centre (-16.1, 29.8) ccw
  line L882 (-16.2174, 28.8586) -> (-17.0653, 28.0624)
  line L883 (-15.9888, 32.8) -> (-15.9888, 31.4975)
  arc A415 (-17.8764, 30.7591) -> (-15.9888, 31.4975) centre (-16.1, 29) ccw
  line L884 (-17.8764, 30.7591) -> (-15.9888, 32.8)
  line L885 (112.3409, -44.4) -> (107.9591, -44.4)
  arc A416 (107.9591, -44.4) -> (107.9591, -53.5) centre (110.15, -48.95) ccw
  line L886 (107.9591, -53.5) -> (112.3364, -53.5)
  line L887 (112.3364, -53.5) -> (112.3364, -53.5022)
  arc A417 (112.3364, -53.5022) -> (114.4671, -46.3299) centre (110.15, -48.95) ccw
  line L888 (114.4671, -46.3299) -> (114.8523, -45.9448)
  line L889 (114.8523, -45.9448) -> (113.1552, -44.2477)
  line L890 (113.1552, -44.2477) -> (112.7701, -44.6329)
  arc A418 (112.7701, -44.6329) -> (112.3409, -44.4) centre (110.15, -48.95) ccw
  circle A419 centre (110.15, -48.95) radius 3.85
  line L891 (-14, -6.9) -> (-19, -6.9)
  line L892 (-19, -6.9) -> (-14, -6.9)
  line L893 (-30.5, -24.9) -> (-25, -24.9)
  line L894 (-25, -24.9) -> (-30.5, -24.9)
  line L895 (-15.9888, 32.8) -> (-15.9888, 31.4975)
  line L896 (-15.9888, 31.4975) -> (-15.9888, 32.8)
  line L897 (-30.5, -13.9) -> (-26, -13.9)
  line L898 (-26, -13.9) -> (-30.5, -13.9)
  line L899 (-19, -1.9) -> (-14, -1.9)
  line L900 (-14, -1.9) -> (-19, -1.9)
  circle A420 centre (110.15, -62.1) radius 0.4
  circle A421 centre (117.6453, -56.4453) radius 2.35
  circle A422 centre (117.6453, -56.4453) radius 5
  arc A423 (-15.4643, 29.0958) -> (-16.2174, 28.8586) centre (-16.1, 29.8) ccw
  arc A424 (-15.4643, 29.0958) -> (-16.2174, 28.8586) centre (-16.1, 29.8) ccw
  line L901 (-25, -13.9) -> (-13, -13.9)
  line L902 (-13, -13.9) -> (-25, -13.9)
  line L903 (-17.0653, 28.0624) -> (-16.4927, 27.4281)
  line L904 (-16.4927, 27.4281) -> (-17.0653, 28.0624)
  circle A425 centre (110.15, -62.1) radius 0.4
  circle A426 centre (110.15, -62.1) radius 2.5
  line L905 (112.3364, -53.5) -> (112.3364, -53.5022)
  line L906 (112.3364, -53.5022) -> (112.3364, -53.5)
  line L907 (-13, -13.9) -> (-13, -7.9)
  line L908 (-13, -7.9) -> (-13, -13.9)
  line L909 (107.9591, -53.5) -> (112.3364, -53.5)
  line L910 (112.3364, -53.5) -> (107.9591, -53.5)
  line L911 (-30.5, -1.9) -> (-26, -1.9)
  line L912 (-26, -1.9) -> (-30.5, -1.9)
  circle A427 centre (-16.1626, -20.3028) radius 0.4
  circle A428 centre (-16.1626, -20.3028) radius 0.4
  line L913 (-20, -1.9) -> (-20, -6.9)
  line L914 (-20, -6.9) -> (-20, -1.9)
  arc A429 (-22.5, 34.3) -> (-31.5, 25.3) centre (-22.5, 25.3) ccw
  arc A430 (-22.5, 34.3) -> (-31.5, 25.3) centre (-22.5, 25.3) ccw
  line L915 (-2.5, 34.3) -> (-2.5, 35.3)
  line L916 (-2.5, 35.3) -> (-2.5, 34.3)
  circle A431 centre (102.6547, -56.4453) radius 5
  circle A432 centre (102.6547, -56.4453) radius 5
  circle A433 centre (117.6453, -56.4453) radius 5
  circle A434 centre (117.6453, -56.4453) radius 5
  line L917 (-16.5461, 27.7924) -> (-16.7087, 27.9725)
  line L918 (-16.7087, 27.9725) -> (-16.5461, 27.7924)
  line L919 (-26, -13.9) -> (-26, -18.9)
  line L920 (-26, -18.9) -> (-26, -13.9)
  line L921 (-31.5, 4.1) -> (-30.5, 4.1)
  line L922 (-30.5, 4.1) -> (-26, 4.1)
  line L923 (-26, 4.1) -> (-25, 4.1)
  line L924 (-25, 4.1) -> (-31.5, 4.1)
  line L925 (-16.7087, 27.9725) -> (-15.4643, 29.0958)
  line L926 (-15.4643, 29.0958) -> (-16.7087, 27.9725)
  arc A435 (-18.6098, -19.7916) -> (-18.6299, -19.9) centre (-16.1626, -20.3028) ccw
  arc A436 (-18.6098, -19.7916) -> (-18.6563, -19.9) centre (-16.3363, -20.8316) ccw
  line L927 (-18.6563, -19.9) -> (-18.6299, -19.9)
  arc A437 (27.2, 10) -> (29.2, 8) centre (29.2, 10) ccw
  arc A438 (27.2, 10) -> (29.2, 8) centre (29.2, 10) ccw
  circle A439 centre (110.15, -62.1) radius 0.4
  circle A440 centre (110.15, -62.1) radius 0.4
  line L928 (-30.5, -18.9) -> (-30.5, -13.9)
  line L929 (-30.5, -13.9) -> (-30.5, -18.9)
  line L930 (-18.6299, -19.9) -> (-18.6563, -19.9)
  line L931 (-18.6563, -19.9) -> (-18.6299, -19.9)
  line L932 (-31.5, 4.1) -> (-32.5, 4.1)
  line L933 (-32.5, 4.1) -> (-31.5, 4.1)
  line L934 (-14, -1.9) -> (-14, -6.9)
  line L935 (-14, -6.9) -> (-14, -1.9)
  line L936 (-26, -18.9) -> (-30.5, -18.9)
  line L937 (-30.5, -18.9) -> (-26, -18.9)
  line L938 (-17.8764, 30.7591) -> (-15.9888, 32.8)
  line L939 (-15.9888, 32.8) -> (-17.8764, 30.7591)
  line L940 (-19, -6.9) -> (-19, -1.9)
  line L941 (-19, -1.9) -> (-19, -6.9)
  arc A441 (107.9591, -44.4) -> (107.9591, -53.5) centre (110.15, -48.95) ccw
  arc A442 (107.9591, -44.4) -> (107.9591, -53.5) centre (110.15, -48.95) ccw
  circle A443 centre (-22.5, 25.3) radius 2.5
  arc A444 (-22, 22.8505) -> (-23, 22.8505) centre (-22.5, 25.3) ccw
  arc A445 (-23, 22.8505) -> (-22, 22.8505) centre (-22.5, 25.3) ccw
  line L942 (-30.5, -6.9) -> (-30.5, -1.9)
  line L943 (-30.5, -1.9) -> (-30.5, -6.9)
  circle A446 centre (-22.5, 25.3) radius 0.4
  circle A447 centre (-22.5, 25.3) radius 0.4
  line L944 (-26, -1.9) -> (-26, -6.9)
  line L945 (-26, -6.9) -> (-26, -1.9)
  line L946 (-26, -18.9) -> (-26, -13.9)
  line L947 (-26, -13.9) -> (-30.5, -13.9)
  line L948 (-30.5, -13.9) -> (-30.5, -18.9)
  line L949 (-30.5, -18.9) -> (-26, -18.9)
  line L950 (-15.2, 27.4281) -> (-16.4927, 27.4281)
  line L951 (-16.4927, 27.4281) -> (-17.0653, 28.0624)
  line L952 (-17.0653, 28.0624) -> (-16.2174, 28.8586)
  arc A448 (-15.4643, 29.0958) -> (-16.2174, 28.8586) centre (-16.1, 29.8) ccw
  line L953 (-15.4643, 29.0958) -> (-16.7087, 27.9725)
  line L954 (-16.7087, 27.9725) -> (-16.5461, 27.7924)
  line L955 (-16.5461, 27.7924) -> (-15.8651, 28.0068)
  arc A449 (-15.6347, 27.9403) -> (-15.8651, 28.0068) centre (-15.8, 27.8) ccw
  line L956 (-15.6347, 27.9403) -> (-15.2, 27.4281)
  line L957 (-25, -24.9) -> (-25, -13.9)
  line L958 (-25, -13.9) -> (-25, -24.9)
  line L959 (-26, -6.9) -> (-30.5, -6.9)
  line L960 (-30.5, -6.9) -> (-26, -6.9)
  line L961 (-21.2419, -66.1) -> (-28.496, -73.3541)
  line L962 (-28.496, -73.3541) -> (-21.2419, -66.1)
  line L963 (-19.5, -38.2) -> (-22.3324, -38.2)
  line L964 (-22.3324, -38.2) -> (-25.5, -38.2)
  line L965 (-25.5, -38.2) -> (-19.5, -38.2)
  line L966 (-21.5816, -73.1909) -> (-27.6189, -73.477)
  line L967 (-27.6189, -73.477) -> (-21.5816, -73.1909)
  arc A450 (46.45, -80.6) -> (47.45, -80.6) centre (46.95, -80.6) ccw
  arc A451 (46.45, -80.6) -> (47.45, -80.6) centre (46.95, -80.6) ccw
  circle A452 centre (-16.25, -62.1) radius 0.4
  line L968 (95.9, -25.9) -> (101.9, -25.9)
  line L969 (101.9, -25.9) -> (101.9, -24.9)
  line L970 (101.9, -24.9) -> (95.9, -24.9)
  line L971 (95.9, -24.9) -> (95.9, -25.9)
  line L972 (-8, -24.9) -> (-2, -24.9)
  line L973 (-2, -24.9) -> (-8, -24.9)
  arc A453 (-30.4722, -66.1) -> (-28.496, -73.3541) centre (-12.5, -65.1) ccw
  arc A454 (-30.4722, -66.1) -> (-28.496, -73.3541) centre (-12.5, -65.1) ccw
  line L974 (-8, -7.9) -> (-8, -24.9)
  line L975 (-8, -24.9) -> (-8, -7.9)
  line L976 (-13, -38.2) -> (-13, -35.3676)
  line L977 (-13, -35.3676) -> (-13, -32.2)
  line L978 (-13, -32.2) -> (-13, -38.2)
  circle A455 centre (102.65, -41.45) radius 3.85
  line L979 (107.185, -39.2283) -> (107.2148, -43.61)
  arc A456 (106.9671, -44.0701) -> (107.2148, -43.61) centre (102.65, -41.45) ccw
  line L980 (106.9671, -44.0701) -> (107.3523, -44.4552)
  line L981 (107.3523, -44.4552) -> (105.6552, -46.1523)
  line L982 (105.6552, -46.1523) -> (105.2701, -45.7671)
  arc A457 (98.115, -43.6717) -> (105.2701, -45.7671) centre (102.65, -41.45) ccw
  line L983 (98.115, -43.6717) -> (98.0852, -39.29)
  arc A458 (107.185, -39.2283) -> (98.0852, -39.29) centre (102.65, -41.45) ccw
  line L984 (-13, -7.9) -> (-8, -7.9)
  line L985 (-8, -7.9) -> (-13, -7.9)
  line L986 (-27.6189, -73.477) -> (-21.2106, -67.0687)
  line L987 (-21.2106, -67.0687) -> (-27.6189, -73.477)
  line L988 (-6.9852, -12.9) -> (-2, -12.9)
  line L989 (-2, -12.9) -> (-2, -7.9)
  line L990 (-2, -7.9) -> (-6.979, -7.9)
  line L991 (-6.979, -7.9) -> (-6.9852, -12.9)
  line L992 (-6.9926, -18.9) -> (-2, -18.9)
  line L993 (-2, -18.9) -> (-2, -13.9)
  line L994 (-2, -13.9) -> (-6.9864, -13.9)
  line L995 (-6.9864, -13.9) -> (-6.9926, -18.9)
  line L996 (114.6448, -36.7477) -> (112.9477, -38.4448)
  line L997 (112.9477, -38.4448) -> (114.6448, -36.7477)
  arc A459 (45.65, -79.6) -> (45.65, -80.6) centre (45.65, -80.1) ccw
  arc A460 (45.65, -79.6) -> (45.65, -80.6) centre (45.65, -80.1) ccw
  arc A461 (-19.5, -35.3676) -> (-22.3324, -38.2) centre (-16.25, -41.45) ccw
  arc A462 (-19.5, -35.3676) -> (-22.3324, -38.2) centre (-16.25, -41.45) ccw
  line L998 (-13, -44.7) -> (-10.1676, -44.7)
  line L999 (-10.1676, -44.7) -> (-7, -44.7)
  line L1000 (-7, -44.7) -> (-13, -44.7)
  circle A463 centre (-16.25, -62.1) radius 0.4
  circle A464 centre (-16.25, -62.1) radius 2.5
  line L1001 (93.9, -27.1) -> (95.9, -27.1)
  line L1002 (95.9, -27.1) -> (93.9, -27.1)
  line L1003 (-12.5, -83.1) -> (-12.5, -78.1)
  line L1004 (-12.5, -78.1) -> (-12.5, -83.1)
  line L1005 (107.2148, -43.61) -> (107.185, -39.2283)
  line L1006 (107.185, -39.2283) -> (107.2148, -43.61)
  circle A465 centre (117.65, -41.45) radius 3.85
  circle A466 centre (117.65, -41.45) radius 3.85
  line L1007 (-19.5, -35.3676) -> (-19.5, -38.2)